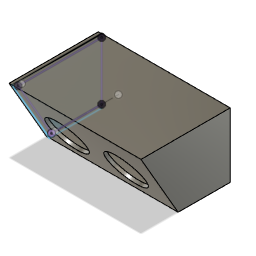
MiniMacroPad v1 (Autodesk Fusion 360 design; units mm, degrees)
Autodesk Fusion 360 part; units mm, degrees
sketch "Sketch1" plane through (0, 0, 0) normal (1, 0, 0) x (0, 0, -1)
  line L0 (0, 0) -> (-20, 34.641)
  line L1 (0, 0) -> (40, 0) construction
  line L2 (-20, 34.641) -> (30, 34.641)
  line L3 (30, 34.641) -> (30, 0)
  line L4 (30, 0) -> (0, 0)
  dimension "d1" = 120
  dimension "d2" = 40
  dimension "d3" = 50
  constraint horizontal L1
  constraint coincident L0.start L1.start
  constraint horizontal L2
  constraint vertical L3
  constraint coincident L1 L3.end
  measures "d1" angle of L0 L1
  measures "d2" distance of L0.start L0.end
  measures "d3" distance of L0.end L2.end
extrude "Extrude1" add sketch "Sketch1" against normal blind 2
sketch "Sketch2" plane through (0, 0, 0) normal (1, 0, 0) x (0, 0, -1)
  line L0 (0, 0) -> (2, 0) construction
  line L1 (30, 0) -> (30, 34.641)
  line L2 (30, 34.641) -> (-20, 34.641)
  line L3 (-20, 34.641) -> (0, 0)
  line L4 (0, 0) -> (30, 0)
  line L5 (-20, 34.641) -> (-18, 34.641) construction
  line L6 (30, 0) -> (30, -2)
  line L7 (30, 34.641) -> (30, 36.641)
  line L8 (30, 36.641) -> (-23.4641, 36.641)
  line L9 (-1.7321, -1) -> (-21.7321, 33.641)
  line L10 (30, -2) -> (0, -1.8905)
  line L11 (-21.7321, 33.641) -> (-23.4641, 36.641)
  line L12 (0, -1.8905) -> (-1.2179, -1.8905)
  line L13 (-1.7321, -1) -> (-1.2179, -1.8905)
  line L14 (30, 0) -> (0, 0)
  line L15 (-20, 34.641) -> (30, 34.641)
  dimension "d7" = 2
  dimension "d10" = 2
  dimension "d12" = 2
  dimension "d13" = 2
  constraint horizontal L0
  constraint coincident L0.start L3.end
  constraint horizontal L5
  constraint coincident L2.end L3.start
  constraint coincident L1.start L4.end
  constraint perpendicular L4 L6
  constraint coincident L1.end L2.start
  constraint perpendicular L2 L7
  constraint perpendicular L7 L8
  constraint coincident L8 L11.end
  constraint coincident L12 L13.end
  measures "d7" distance of L0.start L9.start
  measures "d10" distance of L2.end L9.end
  measures "d12" distance of L1.start L6.end
  measures "d13" distance of L1.end L7.end
extrude "Extrude2" add sketch "Sketch2" against normal blind 2 contours L2 L3 L4 L6 L7 L8 L9 L10 L11 L12 L13 L14 L15
extrude "Extrude3" add sketch "Sketch2" along normal blind 75 contours L2 L3 L4 L6 L7 L8 L9 L10 L11 L12 L13 L14 L15
sketch "Sketch3" plane through (75, 0, 0) normal (1, 0, 0) x (0, 0, -1)
  line L0 (30, 34.641) -> (30, 36.641)
  line L1 (30, 36.641) -> (-23.4641, 36.641)
  line L2 (-23.4641, 36.641) -> (-1.2179, -1.8905)
  line L3 (-1.2179, -1.8905) -> (0, -1.8905)
  line L4 (0, -1.8905) -> (30, -2)
  line L5 (30, -2) -> (30, 0)
  line L6 (-23.4641, 36.641) -> (30, 36.641)
  line L7 (30, -2) -> (-1.2179, -1.8905)
  line L8 (30, 0) -> (0, 0)
  line L9 (0, 0) -> (-20, 34.641)
  line L10 (-20, 34.641) -> (30, 34.641)
  line L11 (30, 34.641) -> (30, 36.641)
  line L12 (30, 36.641) -> (-23.4641, 36.641)
  line L13 (-23.4641, 36.641) -> (-1.2179, -1.8905)
  line L14 (-1.2179, -1.8905) -> (0, -1.8905)
  line L15 (0, -1.8905) -> (30, -2)
  line L16 (30, -2) -> (30, 0)
  line L17 (30, -2) -> (30, 36.641)
  line L18 (30, 36.641) -> (-23.4641, 36.641)
  line L19 (-23.4641, 36.641) -> (-1.2179, -1.8905)
  line L20 (-1.2179, -1.8905) -> (30, -2)
  constraint coincident L1.end L2.start
  constraint coincident L0.end L1.start
  constraint coincident L4.end L5.start
  constraint coincident L2.end L3.start
extrude "Extrude4" add sketch "Sketch3" along normal blind 2 contours L0 L1 L2 L3 L4 L5 L6 L8 L9 L10 L11 L12 L13 L14 L15 L16 L17 L18 L19 | L8 L9 L10 L17
hole "Hole1" at (19.1728, 13.2188, 9.9413) direction (0, 0.5, -0.866025) diameter 24 depth 20 tip angle 118
hole "Hole2" at (54.6679, 13.3913, 10.0409) direction (0, 0.5, -0.866025) diameter 24 depth 20 tip angle 118
